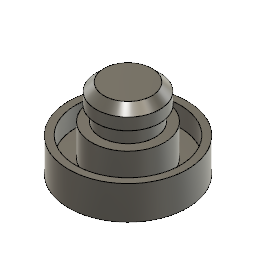
laserCapTop (Autodesk Fusion 360 design; units mm, degrees)
Autodesk Fusion 360 part; units mm, degrees
sketch "Sketch1" plane through (0, 0, 0) normal (0, 1, 0) x (1, 0, 0)
  circle A0 centre (0, 0) radius 15
  dimension "d1" = 30
  measures "d1" diameter of A0
extrude "Extrude1" add sketch "Sketch1" along normal blind 3.5
ref_plane "WorkPlane1" through (0, 3.5, 0) normal (0, 1, 0) x (1, 0, 0)
sketch "Sketch2" plane through (0, 3.5, 0) normal (0, 1, 0) x (1, 0, 0)
  circle A0 centre (0, 0) radius 9.2075
  dimension "d5" = 18.415
  measures "d5" diameter of A0
extrude "Extrude2" add sketch "Sketch2" along normal blind 8
ref_plane "WorkPlane2" through (0, 3.5, 0) normal (0, 1, 0) x (1, 0, 0)
sketch "Sketch3" plane through (0, 3.5, 0) normal (0, 1, 0) x (1, 0, 0)
  circle A0 centre (0, 0) radius 15
  circle A1 centre (0, 0) radius 13.2
  dimension "d9" = 26.4
  measures "d9" diameter of A1
extrude "Extrude3" add sketch "Sketch3" along normal blind 5
ref_plane "WorkPlane3" through (0, 11.5, 0) normal (0, 1, 0) x (1, 0, 0)
sketch "Sketch4" plane through (0, 11.5, 0) normal (0, 1, 0) x (1, 0, 0)
  circle A0 centre (0, 0) radius 6.9
  dimension "d13" = 13.8
  measures "d13" diameter of A0
extrude "Extrude4" add sketch "Sketch4" along normal blind 3.65
ref_plane "WorkPlane4" through (0, 15.15, 0) normal (0, 1, 0) x (1, 0, 0)
sketch "Sketch5" plane through (0, 15.15, 0) normal (0, 1, 0) x (1, 0, 0)
  circle A0 centre (0, 0) radius 8.0538
  dimension "d17" = 16.1075
  measures "d17" diameter of A0
extrude "Extrude5" add sketch "Sketch5" along normal blind 5
chamfer "Chamfer1" distance 2 angle 45 1 edges at (-7.5087, 20.15, 2.9124)
